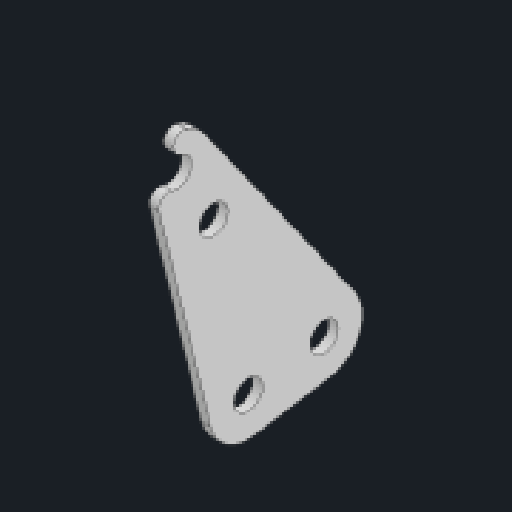
# Autodesk Inventor part: hangPin
Saved by Autodesk Inventor 2024.2 (Build 282272000, 272)
## iProperties
Created: 2024-01-31
Part Number: hangPin
Material: Generic
Document SubType Name: Sheet Metal
Designer: reima
Density: 1 g/cm^3
Sheet Metal Rule: Default
Appearance: Default
Author: reima
Autodesk Inventor part; units mm, degrees
ref_plane "YZ Plane" through (0, 0, 0) normal (1, 0, 0) x (0, 1, 0)
ref_plane "XZ Plane" through (0, 0, 0) normal (0, 1, 0) x (-1, 0, 0)
ref_plane "XY Plane" through (0, 0, 0) normal (0, 0, 1) x (1, 0, 0)
sketch "Sketch1" plane through (0, 0, 0) normal (1, 0, 0) x (0, 1, 0)
  circle A0 centre (-16.5288, 14.8074) radius 3.9624 construction
  circle A1 centre (-54.1655, 3.0444) radius 2.1844 construction
  circle A2 centre (-52.1252, -9.4907) radius 2.1844 construction
  circle A3 centre (-54.1655, 3.0444) radius 2.3495
  circle A4 centre (-52.1252, -9.4907) radius 2.3495
  circle A5 centre (-54.1655, 3.0444) radius 6.35
  circle A6 centre (-52.1252, -9.4907) radius 6.35
  line L0 (-60.433, 2.0242) -> (-58.3927, -10.5108)
  arc A7 (-18.8318, 15.5275) -> (-14.2258, 14.0872) centre (-16.5288, 14.8074) ccw
  line L1 (-16.5288, 14.8074) -> (-18.8318, 15.5275) construction
  line L2 (-16.5288, 14.8074) -> (-14.2258, 14.0872) construction
  arc A8 (-21.8622, 16.475) -> (-11.1955, 13.1397) centre (-16.5288, 14.8074) ccw
  line L3 (-11.1955, 13.1397) -> (-21.8622, 16.475)
  arc A9 (-11.1955, 13.1397) -> (-14.2258, 14.0872) centre (-12.6506, 13.8055) ccw
  arc A10 (-18.8318, 15.5275) -> (-21.8622, 16.475) centre (-20.287, 16.1933) ccw
  line L4 (-20.666, 17.748) -> (-55.6696, 9.2136)
  line L5 (-13.2973, 10.2485) -> (-48.4531, -14.6712)
  circle A11 centre (-26.2996, 8.7467) radius 2.3495
  point P0 (0, 0)
  point P1 (-18.8318, 15.5275)
  dimension "d0" = 4.699
  dimension "d1" = 4.699
  dimension "d4" = 12.7
  dimension "d5" = 12.7
  dimension "d6" = 2.413
  dimension "d7" = 180
  dimension "d8" = 3.175
  dimension "d9" = 1.6002
  dimension "d10" = 1.6002
  dimension "d11" = 4.699
  constraints: 14 point on circle, 12 end point, 9 centre point, 6 tangent, 4 coincident, 2 point on line
  measures "d0" diameter of A3
  measures "d1" diameter of A4
  measures "d4" diameter of A5
  measures "d5" diameter of A6
  measures "d6" radius of A7
  measures "d7" angle of L2 L1
  measures "d8" radial gap between concentric circles of A7 A8
  measures "d9" radius of A9
  measures "d10" radius of A10
  measures "d11" diameter of A11
extrude "Plate1" add sketch "Sketch1" along normal blind 1.5875 contours A5 | A5 L4 A10 A8 L5 A6 | A6 L0 A5 | A6 | A7 L3 A8
sheet face with bend "Face2" sketch "Sketch1" thickness 1.5875 toward (1, 0, 0) bend radius 1.5875 contours A10 L3 | A9 L3
bend "Bend1"
equation "\"d12\" = Thickness"
equation "\"d13\" = BendRadius"
equation "\"d14\" = BendReliefWidth"
equation "\"d16\" = MinimumRemnant"
equation "\"d15\" = BendReliefDepth"
equation "\"d17\" = TransitionRadius"
equation "\"BendRadius\" = Thickness"
equation "\"BendReliefWidth\" = Thickness"
equation "\"BendReliefDepth\" = 0.5 * Thickness"
equation "\"CornerReliefSize\" = 4 * Thickness"
equation "\"MinimumRemnant\" = 2 * Thickness"
equation "\"TransitionRadius\" = BendRadius"
equation "\"JacobiRadiusSize\" = BendRadius"
equation "\"GapSize\" = Thickness"
equation "\"Thickness\" = 1.5875"
body "Solid1"
